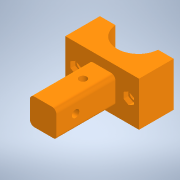
# Autodesk Inventor part: 2_Connettore_inf_sup
Saved by Autodesk Inventor 2020 (Build 240168000, 168)
## iProperties
Created: 2019-10-11
Part Number: 2_Connettore_inf_sup
Material: Generico
Document SubType Name: Modeling
Designer: socci
Density: 1 g/cm^3
Appearance: Arancione
Author: socci
Autodesk Inventor part; units mm, degrees
ref_plane "YZ Plane" through (0, 0, 0) normal (1, 0, 0) x (0, 1, 0)
ref_plane "XZ Plane" through (0, 0, 0) normal (0, 1, 0) x (-1, 0, 0)
ref_plane "XY Plane" through (0, 0, 0) normal (0, 0, 1) x (1, 0, 0)
sketch "Schizzo1" plane through (0, 0, 0) normal (0, 0, 1) x (1, 0, 0)
  line L0 (7, -9) -> (-6, -9)
  line L1 (-9, -6) -> (-9, 6)
  line L2 (-6, 9) -> (6, 9)
  line L3 (9, 6) -> (9, -7)
  arc A0 (7, -9) -> (9, -7) centre (7, -7) ccw
  arc A1 (-9, -6) -> (-6, -9) centre (-6, -6) ccw
  arc A2 (-6, 9) -> (-9, 6) centre (-6, 6) ccw
  arc A3 (9, 6) -> (6, 9) centre (6, 6) ccw
  point P0 (0, 0)
  point P1 (0, 0)
  point P2 (9, -9)
  point P3 (-9, -9)
  point P4 (-9, 9)
  point P5 (9, 9)
  dimension "d0" = 18
  dimension "d44" = 2
  dimension "d45" = 3
  constraints: 8 end point, 8 point on circle, 8 point on line, 8 tangent, 4 centre point, 2 equal radius, 1 coincident, 9 other
  measures "d0" distance of point (-9, 9) point (9, 9)
  measures "d44" radius of A0
  measures "d45" radius of A1
extrude "Estrusione1" add sketch "Schizzo1" along normal blind 40
sketch "Schizzo2" plane through (0, 0, 0) normal (0, 0, -1) x (-1, 0, 0)
  line L0 (25, -15) -> (-25, -15)
  line L1 (-25, -15) -> (-25, 15)
  line L2 (-25, 15) -> (25, 15)
  line L3 (25, 15) -> (25, -15)
  line L4 (25, -15) -> (-25, 15) construction
  line L5 (-25, -15) -> (25, 15) construction
  point P0 (0, 0)
  dimension "d3" = 50
  dimension "d4" = 30
  constraints: 12 end point, 3 midpoint, 2 parallel, 1 horizontal, 1 perpendicular
  measures "d3" distance of L0.start L0.end
  measures "d4" distance of L0.end L1.end
extrude "Estrusione2" add sketch "Schizzo2" along normal blind 23.5
sketch "Schizzo3" plane through (-25, 15, 0) normal (0, 1, 0) x (1, 0, 0)
  circle A0 centre (25, 24.6032) radius 14.5
  point P0 (25, 0)
  dimension "d7" = 29
  constraints: 1 centre point
  measures "d7" diameter of A0
extrude "Estrusione3" cut sketch "Schizzo3" against normal blind 30
sketch "Schizzo4" plane through (0, 0, 0) normal (0, 0, 1) x (1, 0, 0)
  line L0 (-25, -15) -> (-25, 15) projected
  line L1 (-25, 0) -> (-18, 0)
  line L2 (0, 0) -> (-18, 0)
  line L3 (-14.458, 15) -> (-14.458, -15) projected
  line L4 (0, 0) -> (18, 0)
  dimension "d14" = 18
  dimension "d15" = 18
  constraints: 6 end point, 2 horizontal, 1 midpoint, 1 perpendicular
  measures "d14" distance of L2.start L1.end
  measures "d15" distance of L2.start L4.end
hole "Foro1" at (-18, 0, 0) at (18, 0, 0) direction (0, 0, -1) diameter 5 end through all
sketch "Schizzo5" plane through (0, 0, 0) normal (0, 0, 1) x (1, 0, 0)
  circle A0 centre (-18, 0) radius 2.5 projected
  circle A1 centre (18, 0) radius 2.5 projected
  line L0 (-14.5, -2.0207) -> (-18, -4.0415)
  line L1 (-18, -4.0415) -> (-21.5, -2.0207)
  line L2 (-21.5, -2.0207) -> (-21.5, 2.0207)
  line L3 (-21.5, 2.0207) -> (-18, 4.0415)
  line L4 (-18, 4.0415) -> (-14.5, 2.0207)
  line L5 (-14.5, 2.0207) -> (-14.5, -2.0207)
  line L6 (21.5, -2.0207) -> (18, -4.0415)
  line L7 (18, -4.0415) -> (14.5, -2.0207)
  line L8 (14.5, -2.0207) -> (14.5, 2.0207)
  line L9 (14.5, 2.0207) -> (18, 4.0415)
  line L10 (18, 4.0415) -> (21.5, 2.0207)
  line L11 (21.5, 2.0207) -> (21.5, -2.0207)
  point P0 (0, 0)
  point P1 (-14.5, 0)
  point P2 (21.5, 0)
  constraints: 24 end point, 2 coincident, 2 midpoint, 26 other
extrude "Estrusione4" cut sketch "Schizzo5" against normal blind 3.2 contours A0 | A1 | L0 L1 L2 L3 L4 L5 | L6 L7 L8 L9 L10 L11
sketch "Schizzo6" plane through (-9, 9, 40) normal (0, 1, 0) x (1, 0, 0)
  line L0 (9, 40) -> (9, 27)
  line L1 (3, 0) -> (16, 0) projected
  line L2 (9, 40) -> (22, 40) construction
  point P0 (0, 0)
  point P1 (18, 0)
  dimension "d27" = 13
  dimension "d28" = 90
  constraints: 4 end point, 2 perpendicular, 1 horizontal
  measures "d27" distance of L0.start L0.end
  measures "d28" angle of L0 L2
hole "Foro2" at (0, 9, 13) direction (0, -1, 0) diameter 5 end through all
sketch "Schizzo7" plane through (-9, -9, 40) normal (-1, 0, 0) x (0, 0, 1)
  line L0 (0, 2) -> (0, 15) projected
  line L1 (0, 9) -> (-13, 9)
  point P0 (-40, 9)
  point P1 (0, 0)
  point P2 (0, 18)
  dimension "d36" = 13
  constraints: 2 end point, 1 horizontal, 1 point on line
  measures "d36" distance of L1.start L1.end
hole "Foro3" at (-9, 0, 27) direction (1, 0, 0) diameter 5 end through all
